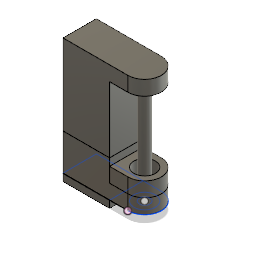
hinge v1 (Autodesk Fusion 360 design; units mm, degrees)
Autodesk Fusion 360 part; units mm, degrees
sketch "Sketch1" plane through (0, 0, 0) normal (0, 1, 0) x (1, 0, 0)
  line L0 (-88.7207, 45.7211) -> (0, 45.7211)
  line L1 (0, 0) -> (-88.7207, 0)
  line L2 (-88.7207, 0) -> (-88.7207, 45.7211)
  arc A0 (0, 0) -> (0, 45.7211) centre (0, 22.8606) ccw
  circle A1 centre (0, 22.8606) radius 14.6792
  circle A2 centre (0, 22.8606) radius 7.1394
  line L3 (-24.9702, 45.7211) -> (-24.9702, 0)
  dimension "d2" = 88.7207
extrude "Extrude5" add sketch "Sketch1" along normal blind 30 contours L0 L1 L2 L3 | L0 L1 A0 L3 makes body 1
extrude "Extrude1" add sketch "Sketch1" along normal blind 20 separate body contours L0 L1 L2 L3 | L0 L1 A0 L3 | A1 | A2 makes body 2
extrude "Extrude2" add sketch "Sketch1" along normal blind 40 contours L0 L1 L2 L3 | A2 bodies 2
ref_plane "WorkPlane1" through (-1.0548, 20, -22.8606) normal (0, 1, 0) x (1, 0, 0)
extrude "Extrude3" add 1 faces at (2.1441, 40, -23.8931) along direction (0, 1, 0) blind 40 on bodies 2 bodies 2
extrude "Extrude4" add 1 faces at (-67.4705, 40, -30.4807) along direction (0, 1, 0) blind 40 on bodies 2 bodies 2
ref_plane "WorkPlane2" through (0, 80, -22.8606) normal (0, 1, 0) x (1, 0, 0)
mirror "Mirror1" about plane through (0, 80, -22.8606) normal (0, 1, 0) of bodies 2 makes body 3
combine "Combine1" operation add target body 3 tool bodies 2
copy_body "Body->Comp1" bodies 3 removing the originals makes body 4 in component "Component"
extrude "Extrude6" add sketch "Sketch1" along normal blind 5 contours L0 L1 L2 L3 bodies 1
extrude "Extrude7" add sketch "Sketch1" against normal blind 10 contours L0 L1 L2 L3 bodies 1
ref_plane "WorkPlane3" through (-32.9301, 15, -22.8606) normal (0, 1, 0) x (1, 0, 0)
mirror "Mirror2" about plane through (-1.0548, 20, -22.8606) normal (0, 1, 0) of bodies 1 makes body 5
combine "Combine2" operation add target body 1 tool bodies 5
copy_body "Body->Comp2" bodies 1 removing the originals makes body 6 in component "Component'"
component "Component" placed x (1, 0, 0) y (0, 1, 0) z (0, 0, 1) at (0, 0, 0)
component "Component'" placed x (1, 0, 0) y (0, 1, 0) z (0, 0, 1) at (0, 0, 0)
